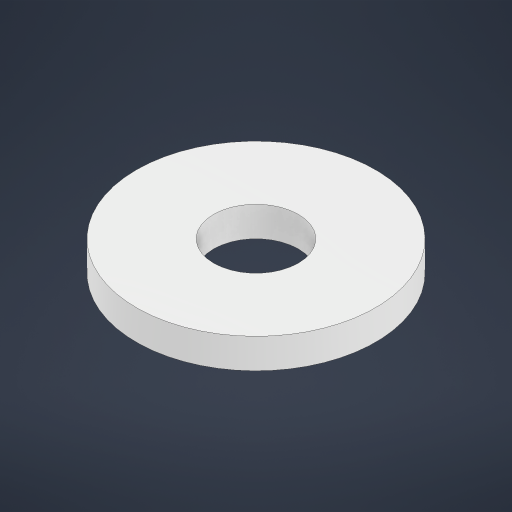
# Autodesk Inventor part: washer
Saved by Autodesk Inventor 2024 (Build 280153000, 153)
## iProperties
Created: 2023-10-29
Part Number: washer
Material: Acetal Resin, White
Document SubType Name: Sheet Metal
Designer: Averey Ku
Density: 1.425 g/cm^3
Appearance: Smooth - White
Flat Pattern Width: 1.27 cm
Flat Pattern Length: 1.27 cm
Flat Pattern Area: 1.6129 cm^2
Sheet Metal Rule: Default_mm
Sheet Metal Width: 0.500 in
Sheet Metal Length: 0.500 in
Sheet Metal Area: 0.250 in^2
Author: Averey Ku
Autodesk Inventor part; units mm, degrees
ref_plane "YZ Plane" through (0, 0, 0) normal (1, 0, 0) x (0, 1, 0)
ref_plane "XZ Plane" through (0, 0, 0) normal (0, 1, 0) x (-1, 0, 0)
ref_plane "XY Plane" through (0, 0, 0) normal (0, 0, 1) x (1, 0, 0)
sketch "Sketch1" plane through (0, 0, 0) normal (0, 1, 0) x (-1, 0, 0)
  circle A0 centre (0, 0) radius 2.2479
  circle A1 centre (0, 0) radius 6.35
  dimension "d0" = 4.4958
  dimension "d1" = 12.7
  constraints: 2 centre point, 2 coincident
  measures "d0" diameter of A0
  measures "d1" diameter of A1
extrude "Extrusion1" add sketch "Sketch1" along normal blind 1.5875
equation "\"BendRadius\" = Thickness"
equation "\"BendReliefWidth\" = Thickness"
equation "\"BendReliefDepth\" = 0.5 * Thickness"
equation "\"CornerReliefSize\" = 4 * Thickness"
equation "\"MinimumRemnant\" = 2 * Thickness"
equation "\"TransitionRadius\" = BendRadius"
equation "\"JacobiRadiusSize\" = BendRadius"
equation "\"GapSize\" = Thickness"
equation "\"Thickness\" = 1.5875"
body "Solid1"
